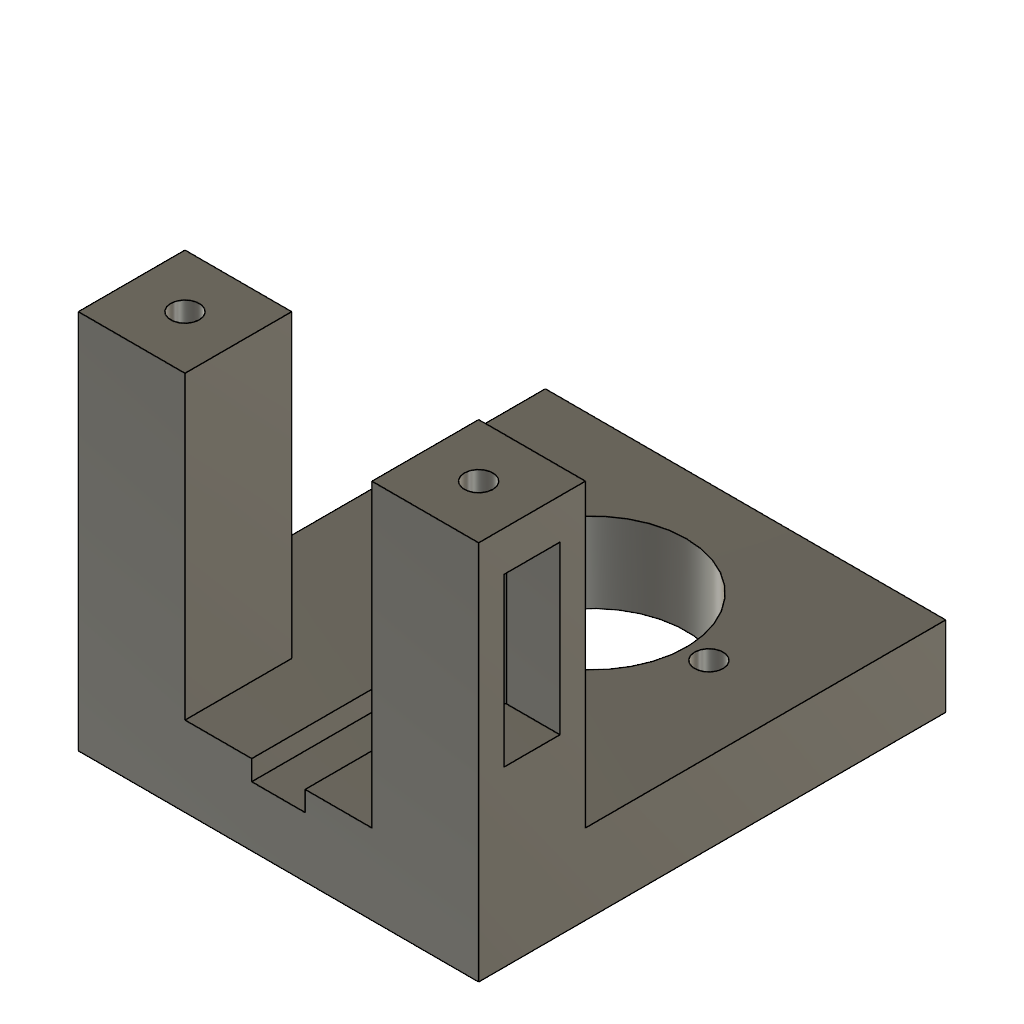
06 - DIFFERENTIAL GEAR MECHANISM (Autodesk Fusion 360 archive; units mm, degrees)
design "05 - PRIMARY SUPPORT MECHANISM ( LEFT SIDE )"
Autodesk Fusion 360 part; units mm, degrees
note: some values were not read from the file. Chosen so that the rebuilt part matches the saved one: which face or edge a step refers to; which pieces of a blend or face edit are solid. Set by a fixed rule: which sketch regions a step uses.
sketch "01 - PRIMARY SUPPORT MECHANISM ( LEFT SIDE ) SKETCH" plane through (0, 0, 0) normal (0, 0, 1) x (1, 0, 0)
  line L0 (0, -35) -> (0, -5.422) construction
  line L1 (13.875, 9.9067) -> (17.5, 7.8138)
  circle A0 centre (17.5, 11.9996) radius 2.14
  line L2 (-13.875, 14.0925) -> (-17.5, 16.1854)
  circle A1 centre (-17.5, 11.9996) radius 2.14
  line L3 (-21.125, 14.0925) -> (-21.125, 9.9067)
  line L4 (4, -5.422) -> (4, -35)
  line L5 (30, 35) -> (30, -35)
  line L6 (-7.6, -5.422) -> (-7.6, 0.1231)
  line L7 (-4, -5.422) -> (-4, -35)
  line L8 (17.5, 7.8138) -> (21.125, 9.9067)
  line L9 (-21.125, 9.9067) -> (-17.5, 7.8138)
  line L10 (7.6, -5.422) -> (7.6, 0.1231)
  line L11 (21.125, 14.0925) -> (17.5, 16.1854)
  line L12 (-30, 35) -> (30, 35)
  line L13 (21.125, 9.9067) -> (21.125, 14.0925)
  line L14 (13.875, 14.0925) -> (13.875, 9.9067)
  line L15 (-17.5, 7.8138) -> (-13.875, 9.9067)
  line L16 (-30, -19) -> (30, -19) construction
  line L17 (30, -35) -> (-30, -35)
  line L18 (17.5, 16.1854) -> (13.875, 14.0925)
  line L19 (-17.5, 11.9996) -> (-17.5, 14.1396) construction
  line L20 (17.5, 11.9996) -> (17.5, 14.1396) construction
  line L21 (-17.5, 11.9996) -> (17.5, 11.9996) construction
  arc A2 (7.6, 0.1231) -> (-7.6, 0.1231) centre (0, 11.9996) ccw
  line L22 (-17.5, 16.1854) -> (-21.125, 14.0925)
  line L23 (-30, -35) -> (-30, 35)
  line L24 (-7.6, -5.422) -> (7.6, -5.422)
  line L25 (-13.875, 9.9067) -> (-13.875, 14.0925)
  point P0 (17.5, 11.9996)
  point P1 (-17.5, 11.9996)
  dimension "d1" = 60
  dimension "d2" = 70
  dimension "d5" = 16
  dimension "d6" = 29.578
  dimension "d7" = 15.2
  dimension "d8" = 5.5451
  dimension "d9" = 14.1
  dimension "d10" = 17.4216
  dimension "d11" = 8
  dimension "d12" = 4
  dimension "d13" = 35
  dimension "d14" = 4.28
  dimension "d15" = 3.625
  dimension "d16" = 4.28
  dimension "d17" = 3.625
  dimension "d19" = 35
  dimension "d20" = 30
  constraint horizontal L12
  constraint vertical L5
  constraint horizontal L17
  constraint vertical L23
  constraint coincident L16.start L23
  constraint coincident L16.end L5
  constraint perpendicular L5 L16
  constraint midpoint L0.start L17
  constraint perpendicular L0 L16
  constraint equal L6 L10
  constraint parallel L6 L10
  constraint perpendicular L10 L24
  constraint coincident L0.end L24
  constraint midpoint L0.end L24
  constraint horizontal L24
  constraint coincident L4.start L24
  constraint coincident L4.end L17
  constraint perpendicular L4 L17
  constraint coincident L7.start L24
  constraint coincident L7.end L17
  constraint perpendicular L7 L17
  constraint horizontal L21
  constraint midpoint A2.centre L21
  constraint coincident P0 A0.centre
  constraint coincident L20.end A0
  constraint perpendicular L20 L21
  constraint coincident L11.end L20
  constraint coincident P1 A1.centre
  constraint coincident L19.end A1
  constraint perpendicular L19 L21
  constraint coincident L2.end L19
  measures "d1" distance of L5.start L12.start
  measures "d2" distance of L12.start L17.end
  measures "d5" distance of L16 L17
  measures "d6" distance of L0.start L0.end
  measures "d7" distance of L10.start L6.start
  measures "d8" distance of L10.end L10.start
  measures "d9" radius of A2
  measures "d10" distance of A2.centre L24
  measures "d11" distance of L4 L7
  measures "d12" distance of L0 L7
  measures "d13" horizontal distance of P1 P0
  measures "d14" diameter of A0
  measures "d15" distance of P0 L13
  measures "d16" diameter of A1
  measures "d17" distance of P1 L15
  measures "d19" distance of origin L12
  measures "d20" distance of origin L23
  measures "d38" distance of L4.start
extrude "Extrude1" add sketch "01 - PRIMARY SUPPORT MECHANISM ( LEFT SIDE ) SKETCH" along normal blind 12 contours L1 L8 L11 L13 L18 A2 | L1 L2 L3 L4 L5 L6 L7 L8 L9 L10 L11 L12 L13 L15 L17 L18 A2 L22 L23 L24 | L2 L3 L9 L15 A2 L22 | A0 | A1
extrude "Extrude2" add sketch "01 - PRIMARY SUPPORT MECHANISM ( LEFT SIDE ) SKETCH" along normal blind 9 contours L4 L7 L17 L24
sketch "02 - PRIMARY SUPPORT MECHANISM ( LEFT SIDE ) SKETCH" plane through (0, 0, 12) normal (0, 0, 1) x (-1, 0, 0)
  line L0 (-4, 5.422) -> (-4, 35)
  line L1 (-4, 35) -> (-30, 35)
  line L2 (-30, 35) -> (-30, -35)
  line L3 (-30, -35) -> (30, -35)
  line L4 (30, -35) -> (30, 35)
  line L5 (30, 35) -> (4, 35)
  line L6 (4, 35) -> (4, 5.422)
  line L7 (4, 5.422) -> (7.6, 5.422)
  line L8 (7.6, 5.422) -> (7.6, -0.1231)
  arc A0 (-7.6, -0.1231) -> (7.6, -0.1231) centre (0, -11.9996) ccw
  line L9 (-7.6, -0.1231) -> (-7.6, 5.422)
  line L10 (-7.6, 5.422) -> (-4, 5.422)
  line L11 (30, 35) -> (4, 35)
  line L12 (-4, 35) -> (-30, 35)
  line L13 (30, 35) -> (14, 35)
  line L14 (-14, 35) -> (-14, 19)
  line L15 (14, 35) -> (14, 19)
  line L16 (-30, 19) -> (-30, 35)
  line L17 (-30, 35) -> (-14, 35)
  line L18 (30, 19) -> (30, 35)
  line L19 (14, 19) -> (30, 19)
  line L20 (-14, 19) -> (-30, 19)
  dimension "d25" = 16
  dimension "d26" = 16
  dimension "d27" = 16
  dimension "d28" = 16
  constraint horizontal L13
  constraint vertical L15
  constraint horizontal L19
  constraint vertical L18
  constraint coincident L4.end L5.start
  constraint horizontal L17
  constraint vertical L14
  constraint horizontal L20
  constraint vertical L16
  constraint coincident L1.end L2.start
  constraint coincident L5.end L6.start
  constraint coincident L0.end L1.start
  measures "d25" distance of L13.end L4.end
  measures "d26" distance of L18.start L4.end
  measures "d27" distance of L14.start L1.end
  measures "d28" distance of L1.end L16.start
extrude "Extrude3" add sketch "02 - PRIMARY SUPPORT MECHANISM ( LEFT SIDE ) SKETCH" along normal blind 45 contours L1 L2 L12 L14 L16 L17 L20 | L4 L5 L11 L13 L15 L18 L19
sketch "03 - PRIMARY SUPPORT MECHANISM ( LEFT SIDE ) SKETCH" plane through (0, 0, 57) normal (0, 0, 1) x (-1, 0, 0)
  line L0 (-14, 19) -> (-14, 35)
  line L1 (-14, 35) -> (-30, 35)
  line L2 (-30, 35) -> (-30, 19)
  line L3 (-30, 19) -> (-14, 19)
  line L4 (-14, 35) -> (-30, 35)
  line L5 (-18.375, 29.0929) -> (-22, 31.1858)
  line L6 (-14, 19) -> (-14, 35)
  line L7 (-22, 22.8142) -> (-18.375, 24.9071)
  line L8 (-14, 27) -> (-30, 27) construction
  line L9 (-25.625, 29.0929) -> (-25.625, 24.9071)
  line L10 (-30, 19) -> (-14, 19)
  line L11 (-22, 23.375) -> (-22, 22.8142)
  line L12 (-25.625, 24.9071) -> (-22, 22.8142)
  line L13 (-22, 22.8142) -> (-30, 22.8142)
  line L14 (-18.375, 24.9071) -> (-18.375, 29.0929)
  line L15 (-22, 31.1858) -> (-22, 30.625)
  line L16 (-30, 31.1858) -> (-30, 22.8142)
  line L17 (-30, 35) -> (-30, 19)
  line L18 (-22, 31.1858) -> (-25.625, 29.0929)
  line L19 (-22, 31.1858) -> (-30, 31.1858)
  circle A0 centre (-22, 27) radius 2.14
  line L20 (-22, 19) -> (-22, 35) construction
  point P0 (-22, 27)
  dimension "d34" = 3.625
  dimension "d35" = 4.28
  dimension "d38" = 16
  dimension "d39" = 16
  constraint midpoint L8.start L6
  constraint midpoint L8.end L17
  constraint midpoint L20.start L10
  constraint midpoint L20.end L4
  constraint midpoint P0 L8
  constraint coincident L5.end L20
  constraint coincident L13.end L17
  constraint perpendicular L13 L17
  constraint coincident L16.start L17
  constraint perpendicular L17 L19
  constraint coincident L11.start L20
  constraint coincident L15.end L20
  constraint coincident P0 A0.centre
  constraint coincident L1.end L2.start
  constraint coincident L0.end L1.start
  constraint coincident L2.end L3.start
  measures "d34" distance of P0 L9
  measures "d35" diameter of A0
  measures "d38" distance of L2.end L0.start
  measures "d39" distance of L0.end L0.start
extrude "Extrude4" cut sketch "03 - PRIMARY SUPPORT MECHANISM ( LEFT SIDE ) SKETCH" against normal blind 25 from surface at -6 contours L2 L9 L12 L13 L16 L17 L18 L19 | L5 L7 L9 L12 L14 L18 | A0
extrude "Extrude5" cut sketch "03 - PRIMARY SUPPORT MECHANISM ( LEFT SIDE ) SKETCH" against normal blind 6 contours A0
sketch "04 - PRIMARY SUPPORT MECHANISM ( LEFT SIDE ) SKETCH" plane through (0, 0, 57) normal (0, 0, 1) x (-1, 0, 0)
  line L0 (14, 19) -> (30, 19)
  line L1 (30, 19) -> (30, 35)
  line L2 (30, 35) -> (14, 35)
  line L3 (14, 35) -> (14, 19)
  line L4 (22, 35) -> (22, 19) construction
  line L5 (30, 27) -> (14, 27) construction
  line L6 (22, 31.1858) -> (18.375, 29.0929)
  line L7 (18.375, 24.9071) -> (22, 22.8142)
  line L8 (30, 35) -> (14, 35)
  line L9 (22, 22.8142) -> (30, 22.8142)
  line L10 (30, 19) -> (30, 35)
  line L11 (25.625, 29.0929) -> (22, 31.1858)
  line L12 (30, 31.1858) -> (30, 22.8142)
  line L13 (22, 22.8142) -> (25.625, 24.9071)
  circle A0 centre (22, 27) radius 2.14
  line L14 (18.375, 29.0929) -> (18.375, 24.9071)
  line L15 (22, 31.1858) -> (30, 31.1858)
  line L16 (25.625, 24.9071) -> (25.625, 29.0929)
  line L17 (14, 19) -> (30, 19)
  line L18 (14, 35) -> (14, 19)
  point P0 (22, 27)
  dimension "d47" = 3.625
  dimension "d48" = 4.28
  dimension "d49" = 16
  dimension "d50" = 16
  constraint midpoint L5.start L10
  constraint midpoint L5.end L18
  constraint midpoint L4.start L8
  constraint midpoint L4.end L17
  constraint midpoint P0 L4
  constraint coincident L6.start L4
  constraint coincident P0 A0.centre
  constraint coincident L9.end L10
  constraint perpendicular L9 L10
  constraint coincident L12.start L10
  constraint perpendicular L10 L15
  constraint coincident L1.end L2.start
  constraint coincident L2.end L3.start
  constraint coincident L0.end L1.start
  measures "d47" distance of P0 L14
  measures "d48" diameter of A0
  measures "d49" distance of L0.end L0.start
  measures "d50" distance of L2.end L0.start
extrude "Extrude6" cut sketch "04 - PRIMARY SUPPORT MECHANISM ( LEFT SIDE ) SKETCH" against normal blind 25 from surface at -6 contours L1 L9 L10 L11 L12 L13 L15 L16 | L6 L7 L11 L13 L14 L16 | A0
extrude "Extrude7" cut sketch "04 - PRIMARY SUPPORT MECHANISM ( LEFT SIDE ) SKETCH" against normal blind 6 contours A0
extrude "Extrude8" cut sketch "01 - PRIMARY SUPPORT MECHANISM ( LEFT SIDE ) SKETCH" along normal blind 12 contours A0 | A1
extrude "Extrude9" cut sketch "01 - PRIMARY SUPPORT MECHANISM ( LEFT SIDE ) SKETCH" along normal blind 4 contours L1 L8 L11 L13 L18 A2 | L2 L3 L9 L15 A2 L22
named bodies: "01 - PRIMARY SUPPORT MECHANISM ( LEFT SIDE )"

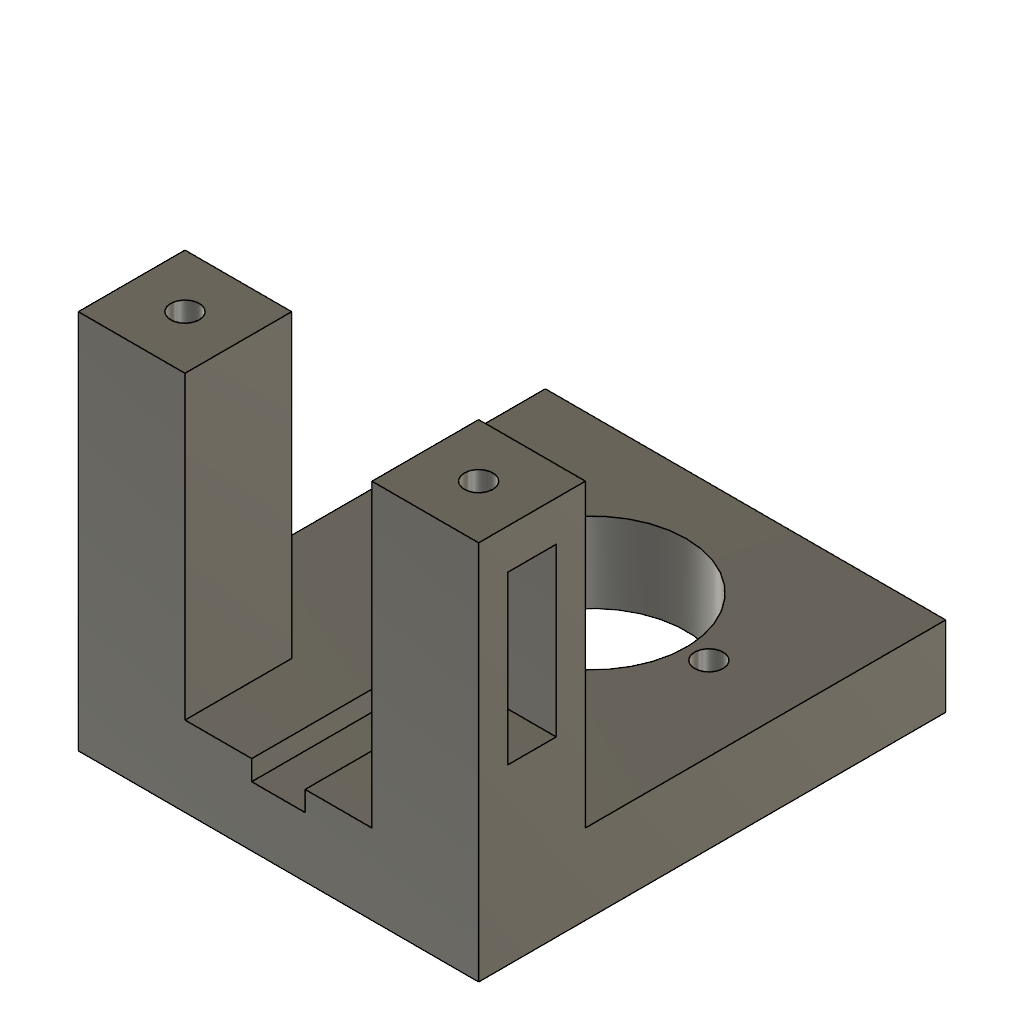
design "04 - PRIMARY SUPPORT MECHANISM ( RIGHT SIDE )"
Autodesk Fusion 360 part; units mm, degrees
sketch "01 - PRIMARY SUPPORT MECHANISM ( RIGHT SIDE ) SKETCH" plane through (0, 0, 0) normal (0, 0, 1) x (1, 0, 0)
  line L0 (-30, 35) -> (30, 35)
  line L1 (30, 35) -> (30, -35)
  line L2 (30, -35) -> (-30, -35)
  line L3 (-30, -35) -> (-30, 35)
  line L4 (-30, -19) -> (30, -19) construction
  line L5 (0, -35) -> (0, -5.422) construction
  line L6 (7.6, -5.422) -> (7.6, 0.1231)
  arc A0 (7.6, 0.1231) -> (-7.6, 0.1231) centre (0, 11.9996) ccw
  line L7 (-7.6, -5.422) -> (7.6, -5.422)
  line L8 (-7.6, -5.422) -> (-7.6, 0.1231)
  line L9 (4, -5.422) -> (4, -35)
  line L10 (-4, -5.422) -> (-4, -35)
  line L11 (-17.5, 11.9996) -> (17.5, 11.9996) construction
  circle A1 centre (17.5, 11.9996) radius 2.14
  line L12 (21.125, 14.0925) -> (17.5, 16.1854)
  line L13 (17.5, 16.1854) -> (13.875, 14.0925)
  line L14 (13.875, 14.0925) -> (13.875, 9.9067)
  line L15 (13.875, 9.9067) -> (17.5, 7.8138)
  line L16 (17.5, 7.8138) -> (21.125, 9.9067)
  line L17 (21.125, 9.9067) -> (21.125, 14.0925)
  line L18 (17.5, 11.9996) -> (17.5, 14.1396) construction
  circle A2 centre (-17.5, 11.9996) radius 2.14
  line L19 (-13.875, 9.9067) -> (-13.875, 14.0925)
  line L20 (-13.875, 14.0925) -> (-17.5, 16.1854)
  line L21 (-17.5, 16.1854) -> (-21.125, 14.0925)
  line L22 (-21.125, 14.0925) -> (-21.125, 9.9067)
  line L23 (-21.125, 9.9067) -> (-17.5, 7.8138)
  line L24 (-17.5, 7.8138) -> (-13.875, 9.9067)
  line L25 (-17.5, 11.9996) -> (-17.5, 14.1396) construction
  point P0 (17.5, 11.9996)
  point P1 (-17.5, 11.9996)
  dimension "d1" = 60
  dimension "d2" = 70
  dimension "d3" = 30
  dimension "d4" = 35
  dimension "d5" = 16
  dimension "d12" = 29.578
  dimension "d14" = 15.2
  dimension "d15" = 5.5451
  dimension "d16" = 14.1
  dimension "d21" = 17.4216
  dimension "d24" = 8
  dimension "d25" = 4
  dimension "d55" = 35
  dimension "d56" = 4.28
  dimension "d57" = 3.625
  dimension "d58" = 4.28
  dimension "d59" = 3.625
  constraint horizontal L0
  constraint vertical L1
  constraint horizontal L2
  constraint vertical L3
  constraint coincident L3 L4.start
  constraint coincident L1 L4.end
  constraint perpendicular L1 L4
  constraint midpoint L2 L5.start
  constraint perpendicular L4 L5
  constraint equal L6 L8
  constraint parallel L6 L8
  constraint perpendicular L6 L7
  constraint coincident L5.end L7
  constraint midpoint L5.end L7
  constraint horizontal L7
  constraint coincident L7 L9.start
  constraint coincident L2 L9.end
  constraint perpendicular L2 L9
  constraint coincident L7 L10.start
  constraint coincident L2 L10.end
  constraint perpendicular L2 L10
  constraint horizontal L11
  constraint midpoint A0.centre L11
  constraint coincident P0 L11.end
  constraint coincident A1 L18.end
  constraint perpendicular L11 L18
  constraint coincident L12.end L18
  constraint coincident P1 L11.start
  constraint coincident A2 L25.end
  constraint perpendicular L11 L25
  constraint coincident L20.end L25
  measures "d1" distance of L0.start L0.end
  measures "d2" distance of L0.start L2.end
  measures "d3" distance of origin L3
  measures "d4" distance of origin L0
  measures "d5" distance of L2 L4
  measures "d12" distance of L5.start L5.end
  measures "d14" distance of L7.start L6.start
  measures "d15" distance of L6.end L6.start
  measures "d16" radius of A0
  measures "d21" distance of A0.centre L7
  measures "d24" distance of L9 L10
  measures "d25" distance of L5 L10
  measures "d55" horizontal distance of P1 P0
  measures "d56" diameter of A1
  measures "d57" distance of P0 L17
  measures "d58" diameter of A2
  measures "d59" distance of P1 L24
extrude "Extrude2" add sketch "01 - PRIMARY SUPPORT MECHANISM ( RIGHT SIDE ) SKETCH" along normal blind 12 contours L0 L1 L2 L3 L6 A0 L7 L8 L9 L10 L12 L13 L15 L16 L17 L20 L21 L22 L23 L24 | A0 L20 L21 L22 L23 L24 | A0 L12 L13 L15 L16 L17 | A1 | A2
extrude "Extrude3" add sketch "01 - PRIMARY SUPPORT MECHANISM ( RIGHT SIDE ) SKETCH" along normal blind 9 contours L2 L7 L9 L10
sketch "02 - PRIMARY SUPPORT MECHANISM ( RIGHT SIDE ) SKETCH" plane through (0, 0, 12) normal (0, 0, 1) x (-1, 0, 0)
  line L0 (7.6, 5.422) -> (7.6, -0.1231)
  arc A0 (-7.6, -0.1231) -> (7.6, -0.1231) centre (0, -11.9996) ccw
  line L1 (-7.6, -0.1231) -> (-7.6, 5.422)
  line L2 (-7.6, 5.422) -> (-4, 5.422)
  line L3 (-4, 5.422) -> (-4, 35)
  line L4 (-4, 35) -> (-30, 35)
  line L5 (-30, 35) -> (-30, -35)
  line L6 (-30, -35) -> (30, -35)
  line L7 (30, -35) -> (30, 35)
  line L8 (30, 35) -> (4, 35)
  line L9 (4, 35) -> (4, 5.422)
  line L10 (4, 5.422) -> (7.6, 5.422)
  line L11 (30, 35) -> (14, 35)
  line L12 (14, 35) -> (14, 19)
  line L13 (14, 19) -> (30, 19)
  line L14 (30, 19) -> (30, 35)
  line L15 (-30, 35) -> (-14, 35)
  line L16 (-14, 35) -> (-14, 19)
  line L17 (-14, 19) -> (-30, 19)
  line L18 (-30, 19) -> (-30, 35)
  dimension "d30" = 16
  dimension "d31" = 16
  dimension "d32" = 16
  dimension "d33" = 16
  constraint horizontal L11
  constraint vertical L12
  constraint horizontal L13
  constraint vertical L14
  constraint coincident L7.end L8.start
  constraint horizontal L15
  constraint vertical L16
  constraint horizontal L17
  constraint vertical L18
  constraint coincident L4.end L5.start
  measures "d30" distance of L7.end L11.end
  measures "d31" distance of L7.end L13.end
  measures "d32" distance of L4.end L15.end
  measures "d33" distance of L4.end L17.end
extrude "Extrude4" add sketch "02 - PRIMARY SUPPORT MECHANISM ( RIGHT SIDE ) SKETCH" along normal blind 45 contours L7 L8 L11 L12 L13 L14 | L4 L5 L15 L16 L17 L18
sketch "03 - PRIMARY SUPPORT MECHANISM ( RIGHT SIDE ) SKETCH" plane through (0, 0, 57) normal (0, 0, 1) x (-1, 0, 0)
  line L0 (-30, 19) -> (-14, 19)
  line L1 (-14, 19) -> (-14, 35)
  line L2 (-14, 35) -> (-30, 35)
  line L3 (-30, 35) -> (-30, 19)
  line L4 (-14, 27) -> (-30, 27) construction
  line L5 (-22, 19) -> (-22, 35) construction
  line L6 (-25.625, 24.9071) -> (-22, 22.8142)
  line L7 (-22, 22.8142) -> (-18.375, 24.9071)
  line L8 (-18.375, 24.9071) -> (-18.375, 29.0929)
  line L9 (-18.375, 29.0929) -> (-22, 31.1858)
  line L10 (-22, 31.1858) -> (-25.625, 29.0929)
  line L11 (-25.625, 29.0929) -> (-25.625, 24.9071)
  line L12 (-22, 22.8142) -> (-30, 22.8142)
  line L13 (-22, 31.1858) -> (-30, 31.1858)
  line L14 (-30, 31.1858) -> (-30, 22.8142)
  circle A0 centre (-22, 27) radius 3.625
  line L15 (-22, 23.375) -> (-22, 22.8142)
  line L16 (-22, 31.1858) -> (-22, 30.625)
  line L17 (-22, 23.375) -> (-30, 23.375)
  line L18 (-22, 30.625) -> (-30, 30.625)
  circle A1 centre (-22, 27) radius 2.14
  point P0 (-22, 27)
  dimension "d36" = 3.625
  dimension "d42" = 4.28
  constraint midpoint L1 L4.start
  constraint midpoint L3 L4.end
  constraint midpoint L0 L5.start
  constraint midpoint L2 L5.end
  constraint midpoint L4 P0
  constraint coincident L5 L9.end
  constraint coincident L3 L12.end
  constraint perpendicular L3 L12
  constraint coincident L3 L13.end
  constraint perpendicular L3 L13
  constraint coincident P0 A0.centre
  constraint tangent L11 A0
  constraint coincident A0 L15.start
  constraint coincident L5 L15.start
  constraint coincident A0 L16.end
  constraint coincident L5 L16.end
  constraint coincident L14 L17.end
  constraint tangent A0 L17
  constraint coincident L14 L18.end
  constraint tangent A0 L18
  measures "d36" distance of P0 L11
  measures "d42" diameter of A1
extrude "Extrude5" cut sketch "03 - PRIMARY SUPPORT MECHANISM ( RIGHT SIDE ) SKETCH" against normal blind 25 from surface at -6 contours L3 L6 L10 L11 L14 L17 L18 | L6 A0 L17 | A0 | L10 A0 L18 | L6 L11 A0 | L10 L11 A0 | A1
extrude "Extrude7" cut sketch "03 - PRIMARY SUPPORT MECHANISM ( RIGHT SIDE ) SKETCH" against normal blind 6 contours A1
sketch "04 - PRIMARY SUPPORT MECHANISM ( RIGHT SIDE ) SKETCH" plane through (0, 0, 57) normal (0, 0, 1) x (-1, 0, 0)
  line L0 (30, 19) -> (30, 35)
  line L1 (30, 35) -> (14, 35)
  line L2 (14, 35) -> (14, 19)
  line L3 (14, 19) -> (30, 19)
  line L4 (30, 27) -> (14, 27) construction
  line L5 (22, 35) -> (22, 19) construction
  line L6 (18.375, 24.9071) -> (22, 22.8142)
  line L7 (22, 22.8142) -> (25.625, 24.9071)
  line L8 (25.625, 24.9071) -> (25.625, 29.0929)
  line L9 (25.625, 29.0929) -> (22, 31.1858)
  line L10 (22, 31.1858) -> (18.375, 29.0929)
  line L11 (18.375, 29.0929) -> (18.375, 24.9071)
  circle A0 centre (22, 27) radius 3.625
  circle A1 centre (22, 27) radius 2.14
  line L12 (22, 22.8142) -> (30, 22.8142)
  line L13 (22, 31.1858) -> (30, 31.1858)
  line L14 (30, 31.1858) -> (30, 22.8142)
  line L15 (22, 23.375) -> (30, 23.375)
  line L16 (22, 30.625) -> (30, 30.625)
  point P0 (22, 27)
  dimension "d45" = 3.625
  dimension "d46" = 4.28
  constraint midpoint L0 L4.start
  constraint midpoint L2 L4.end
  constraint midpoint L1 L5.start
  constraint midpoint L3 L5.end
  constraint midpoint L5 P0
  constraint coincident L5 L9.end
  constraint coincident P0 A0.centre
  constraint tangent L11 A0
  constraint coincident L0 L12.end
  constraint perpendicular L0 L12
  constraint coincident L0 L13.end
  constraint perpendicular L0 L13
  constraint coincident A0 L15.start
  constraint coincident L5 L15.start
  constraint coincident L14 L15.end
  constraint coincident A0 L16.start
  constraint coincident L5 L16.start
  constraint coincident L14 L16.end
  constraint tangent A0 L15
  constraint tangent A0 L16
  measures "d45" distance of P0 L11
  measures "d46" diameter of A1
extrude "Extrude9" cut sketch "04 - PRIMARY SUPPORT MECHANISM ( RIGHT SIDE ) SKETCH" against normal blind 25 from surface at -6 contours L0 L7 L8 L9 L14 L15 L16 | L7 A0 L15 | A0 | L9 A0 L16 | L7 L8 A0 | L8 L9 A0 | A1
extrude "Extrude10" cut sketch "04 - PRIMARY SUPPORT MECHANISM ( RIGHT SIDE ) SKETCH" against normal blind 6 contours A1
extrude "Extrude11" cut sketch "01 - PRIMARY SUPPORT MECHANISM ( RIGHT SIDE ) SKETCH" along normal blind 12 contours A1 | A2
extrude "Extrude12" cut sketch "01 - PRIMARY SUPPORT MECHANISM ( RIGHT SIDE ) SKETCH" along normal blind 4 contours A0 L20 L21 L22 L23 L24 | A0 L12 L13 L15 L16 L17
named bodies: "01 - PRIMARY SUPPORT MECHANISM ( RIGHT SIDE )"

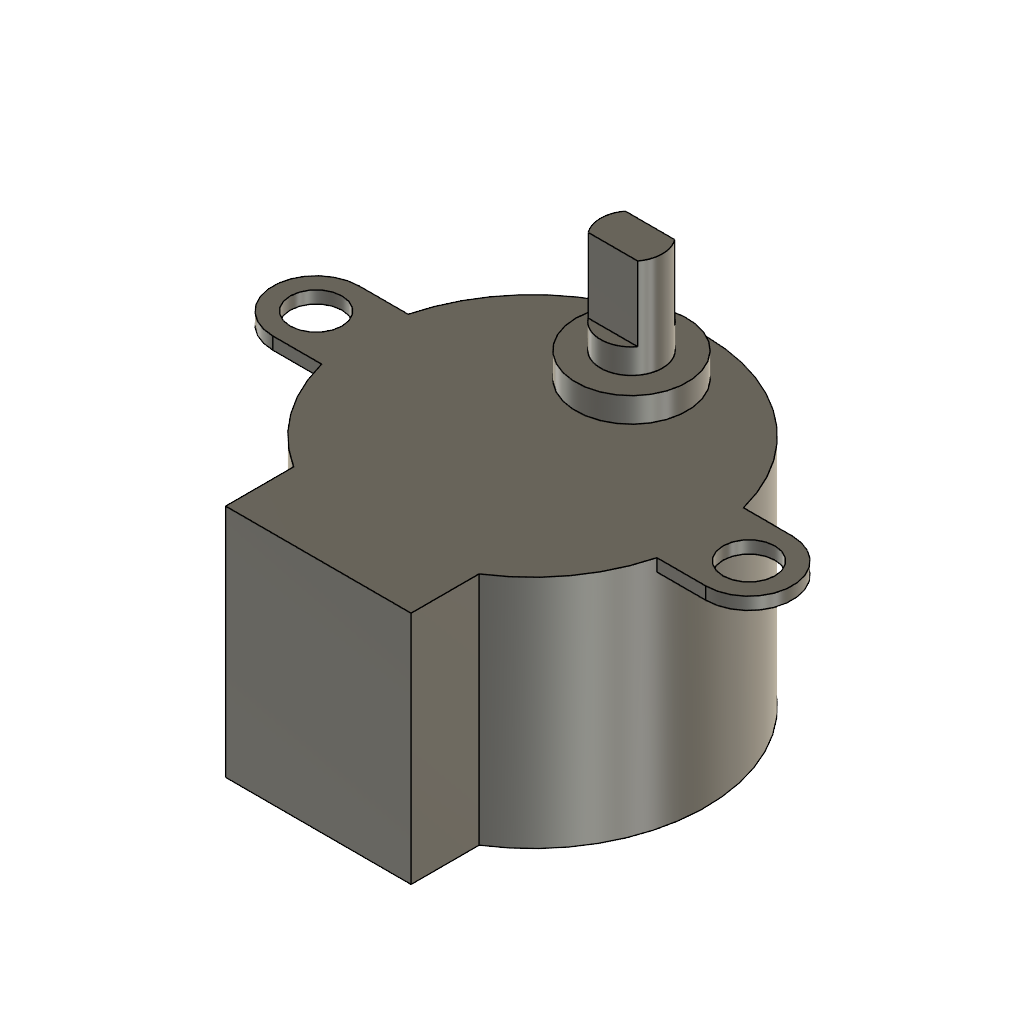
design "03 - 28BYJ-48 STEPPER MOTOR"
Autodesk Fusion 360 part; units mm, degrees
sketch "01 - 28BYJ-48 STEPPER MOTOR BASE SKETCH" plane through (0, 0, 0) normal (0, 0, 1) x (1, 0, 0) in component "01 - 28BYJ-48 STEPPER MOTOR BASE"
  line L0 (-17.5, 0) -> (17.5, 0) construction
  circle A0 centre (-17.5, 0) radius 2.1
  circle A1 centre (17.5, 0) radius 2.1
  arc A2 (-17.5, 3.5) -> (-17.5, -3.5) centre (-17.5, 0) ccw
  arc A3 (17.5, -3.5) -> (17.5, 3.5) centre (17.5, 0) ccw
  line L1 (-17.5, 3.5) -> (-13.5554, 3.5)
  line L2 (13.5554, 3.5) -> (17.5, 3.5)
  line L3 (-17.5, -3.5) -> (-13.5554, -3.5)
  line L4 (13.5554, -3.5) -> (17.5, -3.5)
  line L5 (-7.5, -17.3216) -> (7.5, -17.3216)
  line L6 (7.5, -17.3216) -> (7.5, -11.8216)
  line L7 (-7.5, -17.3216) -> (-7.5, -11.8216)
  line L8 (0, 0) -> (0, 8)
  circle A4 centre (0, 8) radius 4.5
  line L9 (-7.5, -11.8216) -> (-7.5, 0) construction
  line L10 (7.5, -11.8216) -> (7.5, 0) construction
  line L11 (0, -17.3216) -> (0, 0) construction
  line L12 (0, 8) -> (0, 14) construction
  arc A5 (7.5, -11.8216) -> (-7.5, -11.8216) centre (0, 0) ccw
  dimension "d1" = 28
  dimension "d2" = 35
  dimension "d3" = 4.2
  dimension "d4" = 7
  dimension "d5" = 4.2
  dimension "d6" = 7
  dimension "d8" = 15
  dimension "d9" = 8
  dimension "d10" = 9
  dimension "d21" = 5.5
  dimension "d23" = 5.5
  dimension "d36" = 6
  dimension "d37" = 25.3216
  constraint coincident L8.start L11.end
  constraint horizontal L0
  constraint midpoint L8.start L0
  constraint coincident L0.start A0.centre
  constraint concentric A0 A2
  constraint coincident L0.end A1.centre
  constraint concentric A1 A3
  constraint tangent A3 L2
  constraint tangent A2 L1
  constraint tangent A3 L4
  constraint tangent A2 L3
  constraint coincident L1.end A5
  constraint coincident L2.start A5
  constraint collinear L1 L2
  constraint coincident L3.end A5
  constraint coincident L4.start A5
  constraint collinear L3 L4
  constraint perpendicular L5 L6
  constraint perpendicular L5 L7
  constraint perpendicular L0 L8
  constraint coincident L8.end A4.centre
  constraint coincident L0 L9.end
  constraint perpendicular L0 L9
  constraint coincident L0 L10.end
  constraint perpendicular L0 L10
  constraint midpoint L5 L11.start
  constraint perpendicular L0 L11
  constraint coincident L12.end A5
  constraint perpendicular L12 A5
  measures "d1" diameter of A5
  measures "d2" distance of L0.start L0.end
  measures "d3" diameter of A0
  measures "d4" diameter of A2
  measures "d5" diameter of A1
  measures "d6" diameter of A3
  measures "d8" distance of L5.start L5.end
  measures "d9" distance of L8.start L8.end
  measures "d10" diameter of A4
  measures "d21" distance of L5.end L6.end
  measures "d23" distance of L5.start L7.end
  measures "d36" distance of L8.end L12.end
  measures "d37" distance of L5 L8.end
extrude "Extrude1" add sketch "01 - 28BYJ-48 STEPPER MOTOR BASE SKETCH" against normal blind 19 contours L5 L6 L7 A5 | A4 makes body 1 in component "01 - 28BYJ-48 STEPPER MOTOR BASE"
extrude "Extrude2" add sketch "01 - 28BYJ-48 STEPPER MOTOR BASE SKETCH" along normal blind 2 contours A4 bodies 1 in component "01 - 28BYJ-48 STEPPER MOTOR BASE"
extrude "Extrude3" add sketch "01 - 28BYJ-48 STEPPER MOTOR BASE SKETCH" against normal blind 1 contours A2 L1 L3 A5 | A3 L2 L4 A5 bodies 1 in component "01 - 28BYJ-48 STEPPER MOTOR BASE"
extrude "Extrude4" add sketch "01 - 28BYJ-48 STEPPER MOTOR BASE SKETCH" against normal blind 16 contours L5 L6 L7 A5 | A4 bodies 1 in component "01 - 28BYJ-48 STEPPER MOTOR BASE"
sketch "02 - 28BYJ-48 STEPPER MOTOR SHAFT SKETCH" plane through (0, 0, 2) normal (0, 0, 1) x (-1, 0, 0) in component "02 - 28BYJ-48 STEPPER MOTOR SHAFT"
  circle A0 centre (0, -8) radius 4.5
  circle A1 centre (0, -8) radius 2.5
  line L0 (2, -9.5) -> (-2, -9.5)
  line L1 (2, -6.5) -> (-2, -6.5)
  dimension "d24" = 5
  dimension "d25" = 3
  constraint concentric A0 A1
  constraint coincident A1 L0.start
  constraint coincident A1 L0.end
  constraint horizontal L0
  constraint coincident A1 L1.start
  constraint coincident A1 L1.end
  constraint horizontal L1
  constraint equal L0 L1
  measures "d24" diameter of A1
  measures "d25" distance of L0 L1
extrude "Extrude1'" add sketch "02 - 28BYJ-48 STEPPER MOTOR SHAFT SKETCH" along normal blind 2 separate body contours A1 L1 | A1 L0 makes body 2 at (-1.9264, 6.4066, 2.6667) makes body 3 at (0.9832, 10.2985, 3.3333) in component "02 - 28BYJ-48 STEPPER MOTOR SHAFT"
extrude "Extrude2'" add sketch "02 - 28BYJ-48 STEPPER MOTOR SHAFT SKETCH" along normal blind 8 contours A1 L0 L1 bodies 2 3 in component "02 - 28BYJ-48 STEPPER MOTOR SHAFT"
component "01 - 28BYJ-48 STEPPER MOTOR BASE" placed x (1, 0, 0) y (0, 1, 0) z (0, 0, 1) at (0, 0, 0)
component "02 - 28BYJ-48 STEPPER MOTOR SHAFT" placed x (1, 0, 0) y (0, 1, 0) z (0, 0, 1) at (0, 0, 0)
named bodies: "01 - 28BYJ-48 STEPPER MOTOR BASE", "02 - 28BYJ-48 STEPPER MOTOR SHAFT"

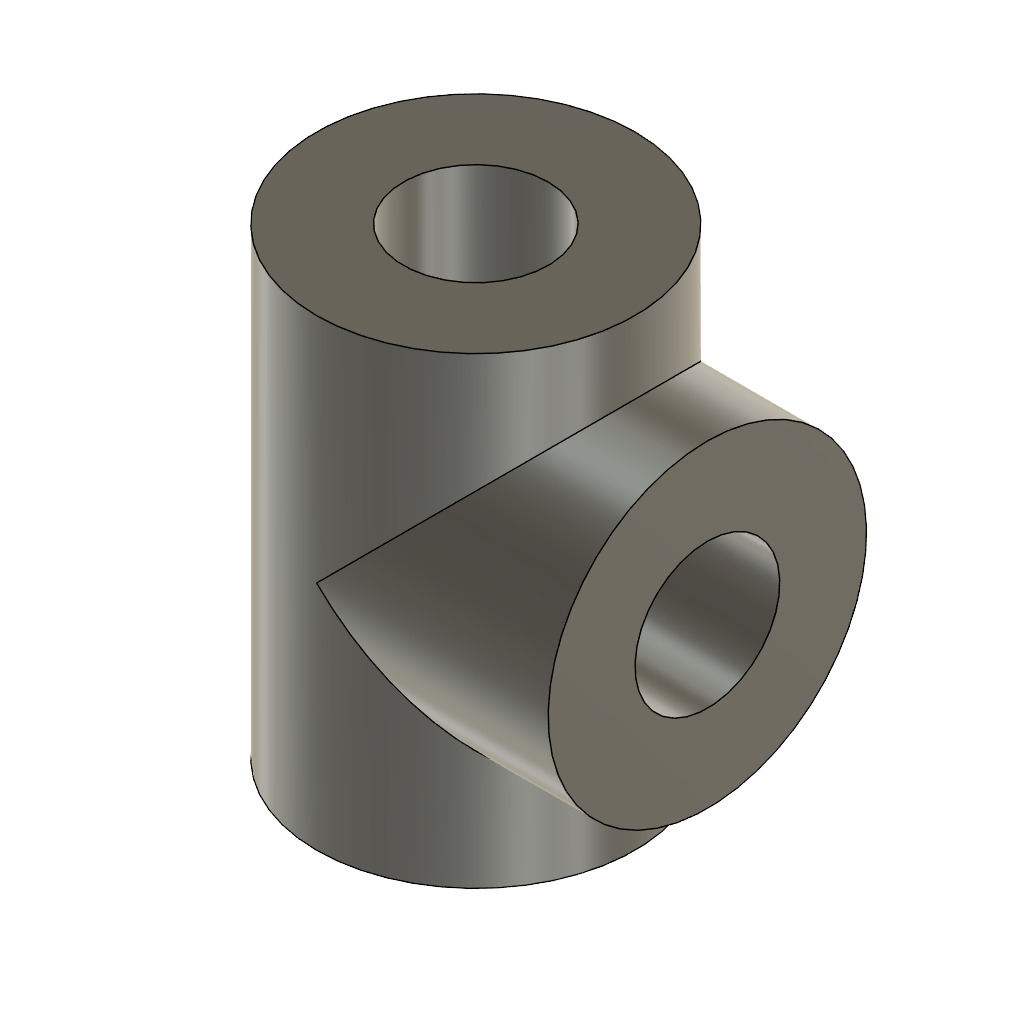
design "02 - T-SHAPE STANDARD EXTERNAL INVOLUTE MITER BEVEL GEAR CONNECTOR"
Autodesk Fusion 360 part; units mm, degrees
sketch "Sketch1" plane through (0, 0, 0) normal (1, 0, 0) x (0, 1, 0) in component "01 - T-SHAPE STANDARD EXTERNAL INVOLUTE MITER BEVEL GEAR CONNECTOR"
  circle A0 centre (0, 0) radius 11
  line L0 (0, 0) -> (0, 11)
  circle A1 centre (0, 0) radius 5
  dimension "d1" = 22
  dimension "d19" = 10
  constraint coincident A0.centre L0.start
  constraint coincident A0 L0.end
  constraint vertical L0
  measures "d1" diameter of A0
  measures "d19" diameter of A1
extrude "Extrude1" add sketch "Sketch1" along normal blind 16 and the other way blind 16 contours A0 | A1 in component "01 - T-SHAPE STANDARD EXTERNAL INVOLUTE MITER BEVEL GEAR CONNECTOR"
ref_plane "WorkPlane2" through (0, 0, 11) normal (0, 0, 1) x (1, 0, 0) in component "01 - T-SHAPE STANDARD EXTERNAL INVOLUTE MITER BEVEL GEAR CONNECTOR"
sketch "Sketch3" plane through (0, 0, 11) normal (0, 0, 1) x (1, 0, 0) in component "01 - T-SHAPE STANDARD EXTERNAL INVOLUTE MITER BEVEL GEAR CONNECTOR"
  circle A0 centre (0, 0) radius 11
  dimension "d13" = 22
  constraint coincident A0.centre origin
  measures "d13" diameter of A0
extrude "Extrude2" add sketch "Sketch3" along normal up to near side of body 1 in component "01 - T-SHAPE STANDARD EXTERNAL INVOLUTE MITER BEVEL GEAR CONNECTOR"
extrude "Extrude3" add 2 faces at (3.1924, -3.1463, 11) (-1.179, 5.1656, 11) along direction (0, 0, 1) blind 5 in component "01 - T-SHAPE STANDARD EXTERNAL INVOLUTE MITER BEVEL GEAR CONNECTOR"
shell "Shell1" thickness 6 removed faces 1 at (5.6593, -1.2423, 16) in component "01 - T-SHAPE STANDARD EXTERNAL INVOLUTE MITER BEVEL GEAR CONNECTOR"
hole "Hole1" at (16, 0, 0) direction (-1, 0, 0) diameter 10 depth 32 tip angle 180 in component "01 - T-SHAPE STANDARD EXTERNAL INVOLUTE MITER BEVEL GEAR CONNECTOR"
component "01 - T-SHAPE STANDARD EXTERNAL INVOLUTE MITER BEVEL GEAR CONNECTOR" placed x (0, 0, -1) y (0, 1, 0) z (1, 0, 0) at (-2.3743, 0, 2.3743)
named bodies: "01 - T-SHAPE STANDARD EXTERNAL INVOLUTE MITER BEVEL GEAR CONNECTOR"
